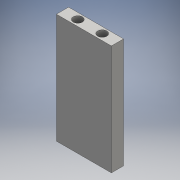
# Autodesk Inventor part: Motor Platform
Saved by Autodesk Inventor 2016 (Build 200138000, 138)
## iProperties
Created: 2015-12-21
Part Number: Motor Platform
Material: Generic
Document SubType Name: Modeling
Designer: jonathan
Density: 1 g/cm^3
Appearance: Default
Author: jonathan
Autodesk Inventor part; units mm, degrees
ref_plane "YZ Plane" through (0, 0, 0) normal (1, 0, 0) x (0, 1, 0)
ref_plane "XZ Plane" through (0, 0, 0) normal (0, 1, 0) x (-1, 0, 0)
ref_plane "XY Plane" through (0, 0, 0) normal (0, 0, 1) x (1, 0, 0)
sketch "Sketch1" plane through (0, 0, 0) normal (0, 1, 0) x (-1, 0, 0)
  line L0 (-45, 90) -> (45, 90)
  line L1 (45, 90) -> (45, -90)
  line L2 (45, -90) -> (-45, -90)
  line L3 (-45, -90) -> (-45, 90)
  line L4 (-45, 90) -> (45, -90) construction
  line L5 (45, 90) -> (-45, -90) construction
  point P0 (0, 0)
  dimension "d0" = 180
  dimension "d1" = 90
  constraints: 12 end point, 2 midpoint, 2 parallel, 1 horizontal, 1 perpendicular
  measures "d0" distance of L0.end L1.end
  measures "d1" distance of L1.end L2.end
extrude "Extrusion1" add sketch "Sketch1" along normal blind 20
sketch "Sketch2" plane through (-45, 0, 90) normal (0, 0, 1) x (1, 0, 0)
  circle A0 centre (65, 10) radius 7.5
  circle A1 centre (25, 10) radius 7.5
  point P0 (45, 0)
  dimension "d4" = 20
  dimension "d5" = 20
  dimension "d6" = 10
  dimension "d7" = 10
  dimension "d8" = 15
  dimension "d9" = 15
  constraints: 2 centre point
  measures "d4" horizontal distance of point (45, 0) A1.centre
  measures "d5" horizontal distance of A0.centre point (45, 0)
  measures "d6" vertical distance of point (45, 0) A1.centre
  measures "d7" vertical distance of point (45, 0) A0.centre
  measures "d8" diameter of A0
  measures "d9" diameter of A1
extrude "Extrusion2" cut sketch "Sketch2" against normal through all
body "Solid1"
